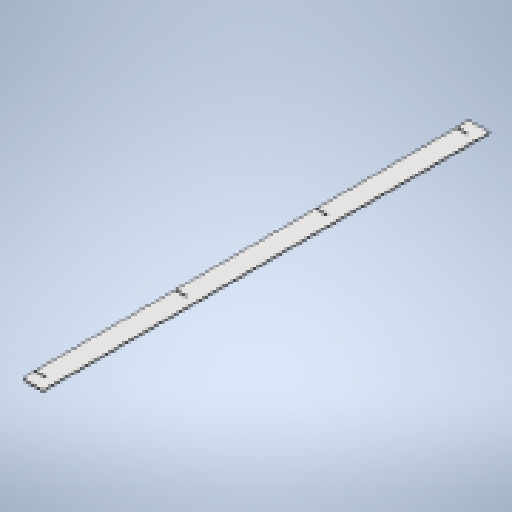
# Autodesk Inventor part: MSC 605 rib cone exit back
Saved by Autodesk Inventor 2025 (Build 290162010, 162A)
## iProperties
Created: 2024-08-26
Part Number: MSC 605 rib cone exit back
Material: Stainless Steel
Document SubType Name: Sheet Metal
Designer: pokla
Density: 8 g/cm^3
Sheet Metal Rule: AISI304 3mm Die 32
Appearance: Default
Stock Number: МОО 605 шпангоут конус выход корма
Mass: 1052.26 g
Surface Area: 935.8 cm^2
Volume: 131.532 cm^3
Flat Pattern Width: 108 cm
Flat Pattern Length: 5 cm
Flat Pattern Area: 540 cm^2
Sheet Metal Width: 1080,000 mm
Sheet Metal Length: 50,000 mm
Sheet Metal Area: 54000,000 mm^2
Author: pokla
Autodesk Inventor part; units mm, degrees
ref_plane "YZ Plane" through (0, 0, 0) normal (1, 0, 0) x (0, 1, 0)
ref_plane "XZ Plane" through (0, 0, 0) normal (0, 1, 0) x (-1, 0, 0)
ref_plane "XY Plane" through (0, 0, 0) normal (0, 0, 1) x (1, 0, 0)
sketch "Sketch1" plane through (0, 0, 0) normal (0, 0, 1) x (1, 0, 0)
  line L0 (-25, 0) -> (25, 0)
  line L1 (25, 0) -> (25, -1080)
  line L2 (25, -1080) -> (-25, -1080)
  line L3 (-25, -1080) -> (-25, 0)
  point P0 (0, 0)
  point P1 (0, 0)
  point P2 (-25, -1153.2713)
  dimension "d0" = 50
  dimension "d1" = 1080
  measures "d0" distance of L0.start L0.end
  measures "d1" distance of L2.end L0.start
extrude "Plate1" add sketch "Sketch1" along normal mid plane 3
sketch "Sketch2" plane through (0, 0, 1.5) normal (0, 0, 1) x (1, 0, 0)
  line L0 (-25, -708.5) -> (1, -708.5)
  line L1 (1, -708.5) -> (1, -711.5)
  line L2 (1, -711.5) -> (-25, -711.5)
  line L3 (-25, -711.5) -> (-25, -708.5)
  line L4 (-25, -1080) -> (-25, 0) projected
  line L5 (-25, -371.5) -> (1, -371.5)
  line L6 (1, -371.5) -> (1, -368.5)
  line L7 (1, -368.5) -> (-25, -368.5)
  line L8 (-25, -368.5) -> (-25, -371.5)
  line L9 (-25, -1048.5) -> (1, -1048.5)
  line L10 (1, -1048.5) -> (1, -1051.5)
  line L11 (1, -1051.5) -> (-25, -1051.5)
  line L12 (-25, -1051.5) -> (-25, -1048.5)
  line L13 (-25, -31.5) -> (1, -31.5)
  line L14 (1, -31.5) -> (1, -28.5)
  line L15 (1, -28.5) -> (-25, -28.5)
  line L16 (-25, -28.5) -> (-25, -31.5)
  point P0 (0, 0)
  point P1 (-25, -710)
  point P2 (-25, -540)
  point P3 (-25, -370)
  point P4 (-25, -540)
  point P5 (-25, -1050)
  point P6 (-25, -30)
  dimension "d15" = 170
  dimension "d16" = 3
  dimension "d17" = 26
  dimension "d18" = 170
  dimension "d19" = 26
  dimension "d20" = 3
  dimension "d23" = 3
  dimension "d24" = 26
  dimension "d25" = 340
  dimension "d26" = 26
  dimension "d27" = 3
  dimension "d29" = 340
  constraints: 32 end point, 8 parallel, 6 midpoint, 4 horizontal, 4 perpendicular, 2 point on line, 2 vertical alignment
  measures "d15" distance of point (-25, -540) point (-25, -710)
  measures "d16" distance of L2.end L0.start
  measures "d17" distance of L1.end L2.end
  measures "d18" distance of point (-25, -370) point (-25, -540)
  measures "d19" distance of L5.start L5.end
  measures "d20" distance of L5.end L6.end
  measures "d23" distance of L11.end L9.start
  measures "d24" distance of L10.end L11.end
  measures "d25" distance of point (-25, -1050) point (-25, -710)
  measures "d26" distance of L13.start L13.end
  measures "d27" distance of L13.end L14.end
  measures "d29" distance of point (-25, -30) point (-25, -370)
extrude "Extrusion1" cut sketch "Sketch2" against normal through all
fillet "Corner Round3" radius 6 2 edges at (-25, -1080, 0) (-25, 0, 0)
sketch "Sketch3" plane through (0, 0, -1.5) normal (0, 0, -1) x (-1, 0, 0)
  line L0 (5.4391, -935.4771) -> (-3.5887, -935.4771) construction
  line L1 (-3.5887, -935.4771) -> (-3.5887, -826.531) construction
  line L2 (-3.5887, -826.531) -> (5.4391, -826.531) construction
  line L3 (5.4391, -826.531) -> (5.4391, -935.4771) construction
  point P0 (0, 0)
  constraints: 2 other
mark "Mark1"
equation "\"d18\" = d15"
equation "\"d20\" = d16"
equation "\"d25\" = 2 * d15"
equation "\"d27\" = d28"
equation "\"d2\" = Thickness"
equation "\"d29\" = d25"
equation "\"BendReliefWidth\" = Thickness"
equation "\"BendReliefDepth\" = 0.5 * Thickness"
equation "\"CornerReliefSize\" = 4 * Thickness"
equation "\"MinimumRemnant\" = 2 * Thickness"
equation "\"TransitionRadius\" = BendRadius"
equation "\"JacobiRadiusSize\" = BendRadius"
equation "\"GapSize\" = Thickness"
equation "\"d28\" = 3"
equation "\"Thickness\" = 3"
equation "\"BendRadius\" = 5"
body "Solid1"
